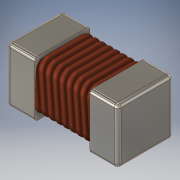
# Autodesk Inventor part: Inductor_1608-Wirewound-0.8mm
Saved by Autodesk Inventor 2018 (Build 220112000, 112)
## iProperties
Created: 2016-08-15
Part Number: Inductor_1608-Wirewound-0.8mm
Material: Copper
Document SubType Name: Modeling
Designer: Bradley
Density: 8.94 g/cm^3
Appearance: Copper - Satin
Author: Bradley
Autodesk Inventor part; units mm, degrees
ref_plane "YZ Plane" through (0, 0, 0) normal (1, 0, 0) x (0, 1, 0)
ref_plane "XZ Plane" through (0, 0, 0) normal (0, 1, 0) x (-1, 0, 0)
sketch "Sketch1" plane through (0, 0, 0) normal (0, 0, 1) x (1, 0, 0)
  line L0 (-0.8, 0.65) -> (-0.4, 0.65)
  line L1 (-0.4, 0.65) -> (-0.4, -0.15)
  line L2 (-0.4, -0.15) -> (-0.8, -0.15)
  line L3 (-0.8, -0.15) -> (-0.8, 0.65)
  line L4 (-0.4, 0.55) -> (0.4, 0.55)
  line L5 (0.4, 0.55) -> (0.4, 0)
  line L6 (0.4, 0) -> (-0.4, 0)
  line L7 (-0.4, 0) -> (-0.4, 0.55)
  line L8 (0.4, 0.65) -> (0.8, 0.65)
  line L9 (0.8, 0.65) -> (0.8, -0.15)
  line L10 (0.8, -0.15) -> (0.4, -0.15)
  line L11 (0.4, -0.15) -> (0.4, 0.65)
  circle A0 centre (-0.445, 0.595) radius 0.045
  circle A1 centre (-0.395, -0.045) radius 0.045
  line L12 (-0.395, -0.045) -> (-0.395, 0)
  point P0 (0, 0)
  point P1 (0, 0.55)
  point P2 (0, 0)
  dimension "d0" = 1.6
  dimension "d1" = 0.8
  dimension "d2" = 0.4
  dimension "d3" = 0.15
  dimension "d6" = 0.1
  dimension "d14" = 0.09
  dimension "d15" = 0.05
  constraints: 26 end point, 6 parallel, 4 horizontal, 4 point on line, 3 perpendicular, 2 collinear, 2 midpoint, 2 tangent, 2 vertical alignment, 1 centre point, 1 coincident, 3 other
  measures "d0" distance between parallel lines of L9 L3
  measures "d1" distance of L2.end L0.start
  measures "d2" distance of L1.end L2.end
  measures "d3" distance between parallel lines of L2 L6
  measures "d6" distance between parallel lines of L4 L0
  measures "d14" diameter of A0
  measures "d15" horizontal distance of L12.start A0.centre
extrude "Extrusion1" add sketch "Sketch1" along normal mid plane 0.8 contours A0 | L0 L1 A1 L2 L3 | A1 L1 | L11 L8 L9 L10 L5
extrude "Extrusion2" add sketch "Sketch1" along normal mid plane 0.6 contours L4 L5 L6 L1
fillet "Fillet1" radius 0.05 20 edges at (-0.6, 0.65, 0.4) (-0.6, 0.65, -0.4) (0, 0.55, -0.3) (0, 0.55, 0.3) (-0.6, -0.15, 0.4) (0, 0, 0.3) (0, 0, -0.3) (-0.6, -0.15, -0.4) (0.6, -0.15, -0.4) (0.6, -0.15, 0.4) (0.6, 0.65, 0.4) (0.8, 0.25, 0.4) (0.8, 0.65, 0) (0.6, 0.65, -0.4) (0.8, 0.25, -0.4) (0.8, -0.15, 0) (-0.8, -0.15, 0) (-0.8, 0.25, 0.4) (-0.8, 0.65, 0) (-0.8, 0.25, -0.4)
ref_plane "Work Plane1" through (-0.445, 0.595, 0) normal (0.9969621, 0.0778877, 0) x (0, 0, 1)
sketch "Sketch5" plane through (-0.445, 0.595, 0) normal (0.9969621, 0.0778877, 0) x (0, 0, 1)
  line L0 (-0.3, 0.0982) -> (-0.3, 0.5468) projected
  ellipse E0 centre (-0.25, 0.5468) end of major axis (-0.2, 0.5468) minor radius 0.0498 (-0.25, 0.5967) -> (-0.3, 0.5468) ccw projected
  line L1 (-0.25, 0.5967) -> (0.25, 0.5967) projected
  ellipse E1 centre (0.25, 0.5468) end of major axis (0.3, 0.5468) minor radius 0.0498 (0.3, 0.5468) -> (0.25, 0.5967) ccw projected
  line L2 (0.3, 0.5468) -> (0.3, 0.0982) projected
  ellipse E2 centre (0.25, 0.0982) end of major axis (0.2, 0.0982) minor radius 0.0498 (0.25, 0.0484) -> (0.3, 0.0982) ccw projected
  line L3 (0.25, 0.0484) -> (-0.25, 0.0484) projected
  ellipse E3 centre (-0.25, 0.0982) end of major axis (-0.3, 0.0982) minor radius 0.0498 (-0.3, 0.0982) -> (-0.25, 0.0484) ccw projected
  ellipse E4 centre (0.35, 0.6964) end of major axis (0.4, 0.6964) minor radius 0.0498 (0.4, 0.6964) -> (0.35, 0.7462) ccw projected
  line L4 (-0.35, 0.7462) -> (0.35, 0.7462) projected
  ellipse E5 centre (-0.35, 0.6964) end of major axis (-0.3, 0.6964) minor radius 0.0498 (-0.35, 0.7462) -> (-0.4, 0.6964) ccw projected
  line L5 (-0.4, -0.0015) -> (-0.4, 0.6964) projected
  ellipse E6 centre (-0.35, -0.0015) end of major axis (-0.4, -0.0015) minor radius 0.0498 (-0.4, -0.0015) -> (-0.35, -0.0513) ccw projected
  line L6 (-0.35, -0.0513) -> (0.35, -0.0513) projected
  ellipse E7 centre (0.35, -0.0015) end of major axis (0.3, -0.0015) minor radius 0.0498 (0.35, -0.0513) -> (0.4, -0.0015) ccw projected
  line L7 (0.4, 0.6964) -> (0.4, -0.0015) projected
  line L8 (0, 0) -> (0.25, 0)
  arc A0 (0.25, 0) -> (0.3482, 0.0982) centre (0.25, 0.0982) ccw
  line L9 (0.3482, 0.0982) -> (0.3482, 0.5468)
  arc A1 (0.3482, 0.5468) -> (0.2255, 0.642) centre (0.25, 0.5468) ccw
  line L10 (0.2255, 0.642) -> (0, 0.642)
  ellipse E8 centre (0.25, 0.5468) end of major axis (0.3, 0.5468) minor radius 0.0498 (0.3, 0.5468) -> (0.25, 0.5967) ccw projected
  point P0 (0, 0.6279)
  constraints: 6 end point, 4 point on circle, 3 tangent, 2 centre point, 1 horizontal, 1 parallel, 1 perpendicular, 11 other
sweep "Sweep1" add profiles "Sketch1" path "Sketch5" path curves L8 A0 L9 A1 L10 contours A0
pattern_circular "Circular Pattern1" count 2 over 360 about axis through (-0.395, -0.045, 0) along (0, 1, 0) of "Sweep1"
pattern_linear "Rectangular Pattern1" count 9 spacing 0.1 along (1, 0, 0) of "Sweep1", "Circular Pattern1"
body "Solid1"
